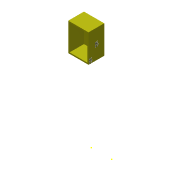
# Autodesk Inventor part: Bucket yellow
Saved by Autodesk Inventor 2015 (Build 190159000, 159)
## iProperties
Created: 2015-04-10
Part Number: Bucket yellow
Material: Generic
Document SubType Name: Modeling
Designer: Vukica
Density: 1 g/cm^3
Appearance: Yellow
Author: Vukica
Autodesk Inventor part; units mm, degrees
ref_plane "YZ Plane" through (0, 0, 0) normal (1, 0, 0) x (0, 1, 0)
ref_plane "XZ Plane" through (0, 0, 0) normal (0, 1, 0) x (-1, 0, 0)
ref_plane "XY Plane" through (0, 0, 0) normal (0, 0, 1) x (1, 0, 0)
ref_plane "Work Plane1" through (220.5144, 586.5816, 98.3522) normal (0, 0, 1) x (1, 0, 0)
sketch "Sketch1" plane through (220.5144, 586.5816, 98.3522) normal (0, 0, 1) x (1, 0, 0)
  line L0 (12.7, 622.3) -> (215.9, 622.3)
  line L1 (12.7, 317.5) -> (215.9, 317.5)
  line L2 (241.3, 317.5) -> (241.3, 596.9)
  line L3 (-12.7, 596.9) -> (-12.7, 317.5)
  line L4 (215.9, 596.9) -> (12.7, 596.9)
  line L5 (215.9, 596.9) -> (215.9, 317.5)
  line L6 (12.7, 317.5) -> (12.7, 596.9)
  line L7 (212.725, 593.725) -> (15.875, 593.725)
  line L8 (15.875, 593.725) -> (15.875, 320.675)
  line L9 (15.875, 320.675) -> (212.725, 320.675)
  line L10 (212.725, 320.675) -> (212.725, 593.725)
  point P0 (-220.5144, -586.5816)
extrude "Extrusion1" add sketch "Sketch1" along normal blind 127 and the other way blind 25.4 contours L10 L9 L8 L7
shell "Shell1" thickness 12.7 removed faces 1 at (302.006, 1089.2899, 225.3522)
sketch "Sketch2" plane through (433.2394, 907.2566, 225.3522) normal (1, 0, 0) x (0, 0, -1)
  line L0 (64.2794, 112.1381) -> (64.2794, 158.5332) construction
  line L1 (64.2794, 158.5332) -> (96.9042, 158.5332) construction
  line L2 (96.9042, 158.5332) -> (96.9042, 112.1381) construction
  line L3 (96.9042, 112.1381) -> (64.2794, 112.1381) construction
  line L4 (3.9697, 3.4317) -> (3.9697, 49.8268) construction
  line L5 (3.9697, 49.8268) -> (36.5945, 49.8268) construction
  line L6 (36.5945, 49.8268) -> (36.5945, 3.4317) construction
  line L7 (36.5945, 3.4317) -> (3.9697, 3.4317) construction
  point P0 (225.3522, -907.2566)
  constraints: 4 other
sketch "Sketch3" plane through (236.3894, 907.2566, 225.3522) normal (-1, 0, 0) x (0, 0, 1)
  line L0 (-63.2632, 158.0563) -> (-63.2632, 111.6612) construction
  line L1 (-63.2632, 111.6612) -> (-95.888, 111.6612) construction
  line L2 (-95.888, 111.6612) -> (-95.888, 158.0563) construction
  line L3 (-95.888, 158.0563) -> (-63.2632, 158.0563) construction
  line L4 (-5.0298, 267.8039) -> (-5.0298, 221.4088) construction
  line L5 (-5.0298, 221.4088) -> (-37.6546, 221.4088) construction
  line L6 (-37.6546, 221.4088) -> (-37.6546, 267.8039) construction
  line L7 (-37.6546, 267.8039) -> (-5.0298, 267.8039) construction
  point P0 (-225.3522, -907.2566)
  constraints: 4 other
body "Solid1"
